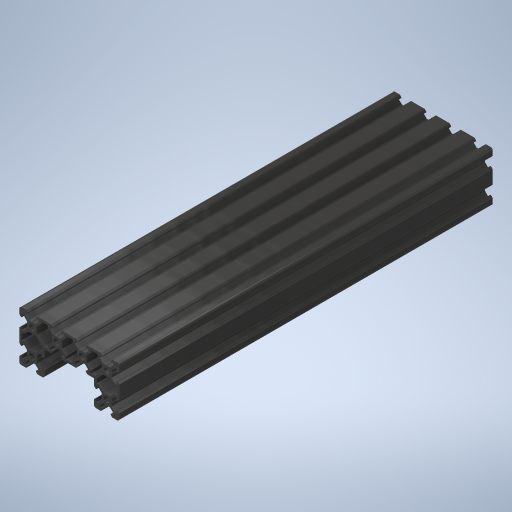
# Autodesk Inventor part: C-Beam 4080 500mm
Saved by Autodesk Inventor 2024.2 (Build 282272000, 272)
## iProperties
Created: 2020-11-22
Part Number: C-Beam 4080 500mm
Material: Aluminum 6061
Document SubType Name: Modeling
Designer: asus
Density: 2.7 g/cm^3
Appearance: Dark Gray
Author: asus
Autodesk Inventor part; units mm, degrees
ref_plane "YZ Plane" through (0, 0, 0) normal (1, 0, 0) x (0, 1, 0)
ref_plane "XZ Plane" through (0, 0, 0) normal (0, 1, 0) x (-1, 0, 0)
ref_plane "XY Plane" through (0, 0, 0) normal (0, 0, 1) x (1, 0, 0)
sketch "Sketch1" plane through (0, 0, 0) normal (0, 0, 1) x (1, 0, 0)
  line L0 (-29.79, -13.9) -> (-30, -13.69)
  line L1 (-30, -13.69) -> (-30.21, -13.9)
  line L2 (-30.21, -13.9) -> (-32.8393, -13.9)
  line L3 (-32.8393, -13.9) -> (-35.5, -16.5607)
  line L4 (-35.5, -16.5607) -> (-35.5, -18.2)
  line L5 (-35.5, -18.2) -> (-33.395, -18.2)
  line L6 (-33.395, -18.2) -> (-33.395, -18.815)
  line L7 (-33.395, -18.815) -> (-34.58, -20)
  line L8 (-34.58, -20) -> (-38.5, -20)
  arc A0 (-40, -18.5) -> (-38.5, -20) centre (-38.5, -18.5) ccw
  line L9 (-40, -18.5) -> (-40, -14.58)
  line L10 (-40, -14.58) -> (-38.815, -13.395)
  line L11 (-38.815, -13.395) -> (-38.2, -13.395)
  line L12 (-38.2, -13.395) -> (-38.2, -15.5)
  line L13 (-38.2, -15.5) -> (-36.5607, -15.5)
  line L14 (-36.5607, -15.5) -> (-33.9, -12.8393)
  line L15 (-33.9, -12.8393) -> (-33.9, -10.21)
  line L16 (-33.9, -10.21) -> (-33.69, -10)
  line L17 (-33.69, -10) -> (-33.9, -9.79)
  line L18 (-33.9, -9.79) -> (-33.9, -7.1607)
  line L19 (-33.9, -7.1607) -> (-36.5607, -4.5)
  line L20 (-36.5607, -4.5) -> (-38.2, -4.5)
  line L21 (-38.2, -4.5) -> (-38.2, -6.605)
  line L22 (-38.2, -6.605) -> (-38.815, -6.605)
  line L23 (-38.815, -6.605) -> (-40, -5.42)
  line L24 (-40, -5.42) -> (-40, 5.42)
  line L25 (-40, 5.42) -> (-38.815, 6.605)
  line L26 (-38.815, 6.605) -> (-38.2, 6.605)
  line L27 (-38.2, 6.605) -> (-38.2, 4.5)
  line L28 (-38.2, 4.5) -> (-36.5607, 4.5)
  line L29 (-36.5607, 4.5) -> (-33.9, 7.1607)
  line L30 (-33.9, 7.1607) -> (-33.9, 9.79)
  line L31 (-33.9, 9.79) -> (-33.69, 10)
  line L32 (-33.69, 10) -> (-33.9, 10.21)
  line L33 (-33.9, 10.21) -> (-33.9, 12.8393)
  line L34 (-33.9, 12.8393) -> (-36.5607, 15.5)
  line L35 (-36.5607, 15.5) -> (-38.2, 15.5)
  line L36 (-38.2, 15.5) -> (-38.2, 13.395)
  line L37 (-38.2, 13.395) -> (-38.815, 13.395)
  line L38 (-38.815, 13.395) -> (-40, 14.58)
  line L39 (-40, 14.58) -> (-40, 18.5)
  arc A1 (-38.5, 20) -> (-40, 18.5) centre (-38.5, 18.5) ccw
  line L40 (-38.5, 20) -> (-34.58, 20)
  line L41 (-34.58, 20) -> (-33.395, 18.815)
  line L42 (-33.395, 18.815) -> (-33.395, 18.2)
  line L43 (-33.395, 18.2) -> (-35.5, 18.2)
  line L44 (-35.5, 18.2) -> (-35.5, 16.5607)
  line L45 (-35.5, 16.5607) -> (-32.8393, 13.9)
  line L46 (-32.8393, 13.9) -> (-30.21, 13.9)
  line L47 (-30.21, 13.9) -> (-30, 13.69)
  line L48 (-30, 13.69) -> (-29.79, 13.9)
  line L49 (-29.79, 13.9) -> (-27.1607, 13.9)
  line L50 (-27.1607, 13.9) -> (-24.5, 16.5607)
  line L51 (-24.5, 16.5607) -> (-24.5, 18.2)
  line L52 (-24.5, 18.2) -> (-26.605, 18.2)
  line L53 (-26.605, 18.2) -> (-26.605, 18.815)
  line L54 (-26.605, 18.815) -> (-25.42, 20)
  line L55 (-25.42, 20) -> (-14.58, 20)
  line L56 (-14.58, 20) -> (-13.395, 18.815)
  line L57 (-13.395, 18.815) -> (-13.395, 18.2)
  line L58 (-13.395, 18.2) -> (-15.5, 18.2)
  line L59 (-15.5, 18.2) -> (-15.5, 16.5607)
  line L60 (-15.5, 16.5607) -> (-12.8393, 13.9)
  line L61 (-12.8393, 13.9) -> (-10.21, 13.9)
  line L62 (-10.21, 13.9) -> (-10, 13.69)
  line L63 (-10, 13.69) -> (-9.79, 13.9)
  line L64 (-9.79, 13.9) -> (-7.1607, 13.9)
  line L65 (-7.1607, 13.9) -> (-4.5, 16.5607)
  line L66 (-4.5, 16.5607) -> (-4.5, 18.2)
  line L67 (-4.5, 18.2) -> (-6.605, 18.2)
  line L68 (-6.605, 18.2) -> (-6.605, 18.815)
  line L69 (-6.605, 18.815) -> (-5.42, 20)
  line L70 (-5.42, 20) -> (5.42, 20)
  line L71 (5.42, 20) -> (6.605, 18.815)
  line L72 (6.605, 18.815) -> (6.605, 18.2)
  line L73 (6.605, 18.2) -> (4.5, 18.2)
  line L74 (4.5, 18.2) -> (4.5, 16.5607)
  line L75 (4.5, 16.5607) -> (7.1607, 13.9)
  line L76 (7.1607, 13.9) -> (9.79, 13.9)
  line L77 (9.79, 13.9) -> (10, 13.69)
  line L78 (10, 13.69) -> (10.21, 13.9)
  line L79 (10.21, 13.9) -> (12.8393, 13.9)
  line L80 (12.8393, 13.9) -> (15.5, 16.5607)
  line L81 (15.5, 16.5607) -> (15.5, 18.2)
  line L82 (15.5, 18.2) -> (13.395, 18.2)
  line L83 (13.395, 18.2) -> (13.395, 18.815)
  line L84 (13.395, 18.815) -> (14.58, 20)
  line L85 (14.58, 20) -> (25.42, 20)
  line L86 (25.42, 20) -> (26.605, 18.815)
  line L87 (26.605, 18.815) -> (26.605, 18.2)
  line L88 (26.605, 18.2) -> (24.5, 18.2)
  line L89 (24.5, 18.2) -> (24.5, 16.5607)
  line L90 (24.5, 16.5607) -> (27.1607, 13.9)
  line L91 (27.1607, 13.9) -> (29.79, 13.9)
  line L92 (29.79, 13.9) -> (30, 13.69)
  line L93 (30, 13.69) -> (30.21, 13.9)
  line L94 (30.21, 13.9) -> (32.8393, 13.9)
  line L95 (32.8393, 13.9) -> (35.5, 16.5607)
  line L96 (35.5, 16.5607) -> (35.5, 18.2)
  line L97 (35.5, 18.2) -> (33.395, 18.2)
  line L98 (33.395, 18.2) -> (33.395, 18.815)
  line L99 (33.395, 18.815) -> (34.58, 20)
  line L100 (34.58, 20) -> (38.5, 20)
  arc A2 (40, 18.5) -> (38.5, 20) centre (38.5, 18.5) ccw
  line L101 (40, 18.5) -> (40, 14.58)
  line L102 (40, 14.58) -> (38.815, 13.395)
  line L103 (38.815, 13.395) -> (38.2, 13.395)
  line L104 (38.2, 13.395) -> (38.2, 15.5)
  line L105 (38.2, 15.5) -> (36.5607, 15.5)
  line L106 (36.5607, 15.5) -> (33.9, 12.8393)
  line L107 (33.9, 12.8393) -> (33.9, 10.21)
  line L108 (33.9, 10.21) -> (33.69, 10)
  line L109 (33.69, 10) -> (33.9, 9.79)
  line L110 (33.9, 9.79) -> (33.9, 7.1607)
  line L111 (33.9, 7.1607) -> (36.5607, 4.5)
  line L112 (36.5607, 4.5) -> (38.2, 4.5)
  line L113 (38.2, 4.5) -> (38.2, 6.605)
  line L114 (38.2, 6.605) -> (38.815, 6.605)
  line L115 (38.815, 6.605) -> (40, 5.42)
  line L116 (40, 5.42) -> (40, -5.42)
  line L117 (40, -5.42) -> (38.815, -6.605)
  line L118 (38.815, -6.605) -> (38.2, -6.605)
  line L119 (38.2, -6.605) -> (38.2, -4.5)
  line L120 (38.2, -4.5) -> (36.5607, -4.5)
  line L121 (36.5607, -4.5) -> (33.9, -7.1607)
  line L122 (33.9, -7.1607) -> (33.9, -9.79)
  line L123 (33.9, -9.79) -> (33.69, -10)
  line L124 (33.69, -10) -> (33.9, -10.21)
  line L125 (33.9, -10.21) -> (33.9, -12.8393)
  line L126 (33.9, -12.8393) -> (36.5607, -15.5)
  line L127 (36.5607, -15.5) -> (38.2, -15.5)
  line L128 (38.2, -15.5) -> (38.2, -13.395)
  line L129 (38.2, -13.395) -> (38.815, -13.395)
  line L130 (38.815, -13.395) -> (40, -14.58)
  line L131 (40, -14.58) -> (40, -18.5)
  arc A3 (38.5, -20) -> (40, -18.5) centre (38.5, -18.5) ccw
  line L132 (38.5, -20) -> (34.58, -20)
  line L133 (34.58, -20) -> (33.395, -18.815)
  line L134 (33.395, -18.815) -> (33.395, -18.2)
  line L135 (33.395, -18.2) -> (35.5, -18.2)
  line L136 (35.5, -18.2) -> (35.5, -16.5607)
  line L137 (35.5, -16.5607) -> (32.8393, -13.9)
  line L138 (32.8393, -13.9) -> (30.21, -13.9)
  line L139 (30.21, -13.9) -> (30, -13.69)
  line L140 (30, -13.69) -> (29.79, -13.9)
  line L141 (29.79, -13.9) -> (27.1607, -13.9)
  line L142 (27.1607, -13.9) -> (24.5, -16.5607)
  line L143 (24.5, -16.5607) -> (24.5, -18.2)
  line L144 (24.5, -18.2) -> (26.605, -18.2)
  line L145 (26.605, -18.2) -> (26.605, -18.815)
  line L146 (26.605, -18.815) -> (25.42, -20)
  line L147 (25.42, -20) -> (21.5, -20)
  arc A4 (20, -18.5) -> (21.5, -20) centre (21.5, -18.5) ccw
  line L148 (20, -18.5) -> (20, -14.58)
  line L149 (20, -14.58) -> (21.185, -13.395)
  line L150 (21.185, -13.395) -> (21.8, -13.395)
  line L151 (21.8, -13.395) -> (21.8, -15.5)
  line L152 (21.8, -15.5) -> (23.4393, -15.5)
  line L153 (23.4393, -15.5) -> (26.1, -12.8393)
  line L154 (26.1, -12.8393) -> (26.1, -10.21)
  line L155 (26.1, -10.21) -> (26.31, -10)
  line L156 (26.31, -10) -> (26.1, -9.79)
  line L157 (26.1, -9.79) -> (26.1, -7.1607)
  line L158 (26.1, -7.1607) -> (23.4393, -4.5)
  line L159 (23.4393, -4.5) -> (21.8, -4.5)
  line L160 (21.8, -4.5) -> (21.8, -6.605)
  line L161 (21.8, -6.605) -> (21.185, -6.605)
  line L162 (21.185, -6.605) -> (20, -5.42)
  line L163 (20, -5.42) -> (20, 0)
  line L164 (20, 0) -> (14.58, 0)
  line L165 (14.58, 0) -> (13.395, 1.185)
  line L166 (13.395, 1.185) -> (13.395, 1.8)
  line L167 (13.395, 1.8) -> (15.5, 1.8)
  line L168 (15.5, 1.8) -> (15.5, 3.4393)
  line L169 (15.5, 3.4393) -> (12.8393, 6.1)
  line L170 (12.8393, 6.1) -> (10.21, 6.1)
  line L171 (10.21, 6.1) -> (10, 6.31)
  line L172 (10, 6.31) -> (9.79, 6.1)
  line L173 (9.79, 6.1) -> (7.1607, 6.1)
  line L174 (7.1607, 6.1) -> (4.5, 3.4393)
  line L175 (4.5, 3.4393) -> (4.5, 1.8)
  line L176 (4.5, 1.8) -> (6.605, 1.8)
  line L177 (6.605, 1.8) -> (6.605, 1.185)
  line L178 (6.605, 1.185) -> (5.42, 0)
  line L179 (5.42, 0) -> (-5.42, 0)
  line L180 (-5.42, 0) -> (-6.605, 1.185)
  line L181 (-6.605, 1.185) -> (-6.605, 1.8)
  line L182 (-6.605, 1.8) -> (-4.5, 1.8)
  line L183 (-4.5, 1.8) -> (-4.5, 3.4393)
  line L184 (-4.5, 3.4393) -> (-7.1607, 6.1)
  line L185 (-7.1607, 6.1) -> (-9.79, 6.1)
  line L186 (-9.79, 6.1) -> (-10, 6.31)
  line L187 (-10, 6.31) -> (-10.21, 6.1)
  line L188 (-10.21, 6.1) -> (-12.8393, 6.1)
  line L189 (-12.8393, 6.1) -> (-15.5, 3.4393)
  line L190 (-15.5, 3.4393) -> (-15.5, 1.8)
  line L191 (-15.5, 1.8) -> (-13.395, 1.8)
  line L192 (-13.395, 1.8) -> (-13.395, 1.185)
  line L193 (-13.395, 1.185) -> (-14.58, 0)
  line L194 (-14.58, 0) -> (-20, 0)
  line L195 (-20, 0) -> (-20, -5.42)
  line L196 (-20, -5.42) -> (-21.185, -6.605)
  line L197 (-21.185, -6.605) -> (-21.8, -6.605)
  line L198 (-21.8, -6.605) -> (-21.8, -4.5)
  line L199 (-21.8, -4.5) -> (-23.4393, -4.5)
  line L200 (-23.4393, -4.5) -> (-26.1, -7.1607)
  line L201 (-26.1, -7.1607) -> (-26.1, -9.79)
  line L202 (-26.1, -9.79) -> (-26.31, -10)
  line L203 (-26.31, -10) -> (-26.1, -10.21)
  line L204 (-26.1, -10.21) -> (-26.1, -12.8393)
  line L205 (-26.1, -12.8393) -> (-23.4393, -15.5)
  line L206 (-23.4393, -15.5) -> (-21.8, -15.5)
  line L207 (-21.8, -15.5) -> (-21.8, -13.395)
  line L208 (-21.8, -13.395) -> (-21.185, -13.395)
  line L209 (-21.185, -13.395) -> (-20, -14.58)
  line L210 (-20, -14.58) -> (-20, -18.5)
  arc A5 (-21.5, -20) -> (-20, -18.5) centre (-21.5, -18.5) ccw
  line L211 (-21.5, -20) -> (-25.42, -20)
  line L212 (-25.42, -20) -> (-26.605, -18.815)
  line L213 (-26.605, -18.815) -> (-26.605, -18.2)
  line L214 (-26.605, -18.2) -> (-24.5, -18.2)
  line L215 (-24.5, -18.2) -> (-24.5, -16.5607)
  line L216 (-24.5, -16.5607) -> (-27.1607, -13.9)
  line L217 (-27.1607, -13.9) -> (-29.79, -13.9)
  line L218 (2.7, 16.2393) -> (2.7, 18.2)
  line L219 (2.7, 18.2) -> (-2.7, 18.2)
  line L220 (-2.7, 18.2) -> (-2.7, 16.2393)
  line L221 (-2.7, 16.2393) -> (-6.1, 12.8393)
  line L222 (-6.1, 12.8393) -> (-6.1, 7.1607)
  line L223 (-6.1, 7.1607) -> (-2.7, 3.7607)
  line L224 (-2.7, 3.7607) -> (-2.7, 1.8)
  line L225 (-2.7, 1.8) -> (2.7, 1.8)
  line L226 (2.7, 1.8) -> (2.7, 3.7607)
  line L227 (2.7, 3.7607) -> (6.1, 7.1607)
  line L228 (6.1, 7.1607) -> (6.1, 12.8393)
  line L229 (6.1, 12.8393) -> (2.7, 16.2393)
  line L230 (-17.3, 16.2393) -> (-17.3, 18.2)
  line L231 (-17.3, 18.2) -> (-22.7, 18.2)
  line L232 (-22.7, 18.2) -> (-22.7, 16.2393)
  line L233 (-22.7, 16.2393) -> (-26.1, 12.8393)
  line L234 (-26.1, 12.8393) -> (-26.1, 7.1607)
  line L235 (-26.1, 7.1607) -> (-20.7393, 1.8)
  line L236 (-20.7393, 1.8) -> (-17.3, 1.8)
  line L237 (-17.3, 1.8) -> (-17.3, 3.7607)
  line L238 (-17.3, 3.7607) -> (-13.9, 7.1607)
  line L239 (-13.9, 7.1607) -> (-13.9, 12.8393)
  line L240 (-13.9, 12.8393) -> (-17.3, 16.2393)
  line L241 (36.2393, -2.7) -> (38.2, -2.7)
  line L242 (38.2, -2.7) -> (38.2, 2.7)
  line L243 (38.2, 2.7) -> (36.2393, 2.7)
  line L244 (36.2393, 2.7) -> (32.8393, 6.1)
  line L245 (32.8393, 6.1) -> (27.1607, 6.1)
  line L246 (27.1607, 6.1) -> (21.8, 0.7393)
  line L247 (21.8, 0.7393) -> (21.8, -2.7)
  line L248 (21.8, -2.7) -> (23.7607, -2.7)
  line L249 (23.7607, -2.7) -> (27.1607, -6.1)
  line L250 (27.1607, -6.1) -> (32.8393, -6.1)
  line L251 (32.8393, -6.1) -> (36.2393, -2.7)
  line L252 (22.7, 16.2393) -> (22.7, 18.2)
  line L253 (22.7, 18.2) -> (17.3, 18.2)
  line L254 (17.3, 18.2) -> (17.3, 16.2393)
  line L255 (17.3, 16.2393) -> (13.9, 12.8393)
  line L256 (13.9, 12.8393) -> (13.9, 7.1607)
  line L257 (13.9, 7.1607) -> (17.3, 3.7607)
  line L258 (17.3, 3.7607) -> (17.3, 1.8)
  line L259 (17.3, 1.8) -> (20.7393, 1.8)
  line L260 (20.7393, 1.8) -> (26.1, 7.1607)
  line L261 (26.1, 7.1607) -> (26.1, 12.8393)
  line L262 (26.1, 12.8393) -> (22.7, 16.2393)
  line L263 (-36.2393, 2.7) -> (-38.2, 2.7)
  line L264 (-38.2, 2.7) -> (-38.2, -2.7)
  line L265 (-38.2, -2.7) -> (-36.2393, -2.7)
  line L266 (-36.2393, -2.7) -> (-32.8393, -6.1)
  line L267 (-32.8393, -6.1) -> (-27.1607, -6.1)
  line L268 (-27.1607, -6.1) -> (-23.7607, -2.7)
  line L269 (-23.7607, -2.7) -> (-21.8, -2.7)
  line L270 (-21.8, -2.7) -> (-21.8, 0.7393)
  line L271 (-21.8, 0.7393) -> (-27.1607, 6.1)
  line L272 (-27.1607, 6.1) -> (-32.8393, 6.1)
  line L273 (-32.8393, 6.1) -> (-36.2393, 2.7)
  circle A6 centre (10, 10) radius 2.3
  circle A7 centre (-10, 10) radius 2.3
  circle A8 centre (-30, 10) radius 2.3
  circle A9 centre (-30, -10) radius 2.3
  circle A10 centre (30, -10) radius 2.3
  circle A11 centre (30, 10) radius 2.3
  circle A12 centre (-30, -10) radius 2.5
  circle A13 centre (-10, 10) radius 2.5
  circle A14 centre (10, 10) radius 2.5
  circle A15 centre (30, -10) radius 2.5
  point P0 (0, 0)
  point P1 (0, 0)
  constraints: 548 end point, 16 centre point, 12 point on circle, 1 midpoint
extrude "Extrusion1" add sketch "Sketch1" along normal blind 300 contours L0 L1 L2 L3 L4 L5 L6 L7 L8 A0 L9 L10 L11 L12 L13 L14 L15 L16 L17 L18 L19 L20 L21 L22 L23 L24 L25 L26 L27 L28 L29 L30 L31 L32 L33 L34 L35 L36 L37 L38 L39 A1 L40 L41 L42 L43 L44 L45 L46 L47 L48 L49 L50 L51 L52 L53 L54 L55 L56 L57 L58 L59 L60 L61 L62 L63 L64 L65 L66 L67 L68 L69 L70 L71 L72 L73 L74 L75 L76 L77 L78 L79 L80 L81 L82 L83 L84 L85 L86 L87 L88 L89 L90 L91 L92 L93 L94 L95 L96 L97 L98 L99 L100 A2 L101 L102 L103 L104 L105 L106 L107 L108 L109 L110 L111 L112 L113 L114 L115 L116 L117 L118 L119 L120 L121 L122 L123 L124 L125 L126 L127 L128 L129 L130 L131 A3 L132 L133 L134 L135 L136 L137 L138 L139 L140 L141 L142 L143 L144 L145 L146 L147 A4 L148 L149 L150 L151 L152 L153 L154 L155 L156 L157 L158 L159 L160 L161 L162 L163 L164 L165 L166 L167 L168 L169 L170 L171 L172 L173 L174 L175 L176 L177 L178 L179 L180 L181 L182 L183 L184 L185 L186 L187 L188 L189 L190 L191 L192 L193 L194 L195 L196 L197 L198 L199 L200 L201 L202 L203 L204 L205 L206 L207 L208 L209 L210 A5 L211 L212 L213 L214 L215 L216 L217
body "Solid1"
